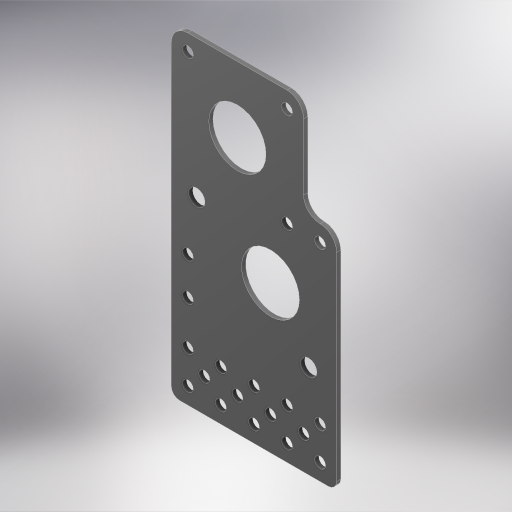
# Autodesk Inventor part: POM 1
Saved by Autodesk Inventor 2024 (Build 280153000, 153)
## iProperties
Created: 2023-09-01
Part Number: POM 1
Material: Acetal Resin, Black
Document SubType Name: Modeling
Designer: aaron
Density: 1.425 g/cm^3
Appearance: Smooth - Black
Author: aaron
Autodesk Inventor part; units mm, degrees
ref_plane "YZ Plane" through (0, 0, 0) normal (1, 0, 0) x (0, 1, 0)
ref_plane "XZ Plane" through (0, 0, 0) normal (0, 1, 0) x (-1, 0, 0)
ref_plane "XY Plane" through (0, 0, 0) normal (0, 0, 1) x (1, 0, 0)
sketch "Sketch1" plane through (0, 0, 0) normal (0, 0, 1) x (1, 0, 0)
  line L0 (57.15, -58.7375) -> (-57.15, -58.7375)
  line L1 (-57.15, -58.7375) -> (-57.15, 58.7375)
  line L2 (-57.15, 58.7375) -> (57.15, 58.7375)
  line L3 (57.15, 58.7375) -> (57.15, -58.7375)
  line L4 (57.15, -58.7375) -> (-57.15, 58.7375) construction
  line L5 (-57.15, -58.7375) -> (57.15, 58.7375) construction
  line L6 (-57.15, 58.7375) -> (-19.05, 58.7375)
  line L7 (-19.05, 58.7375) -> (-19.05, 20.6375)
  line L8 (-19.05, 20.6375) -> (-57.15, 20.6375)
  line L9 (-57.15, 20.6375) -> (-57.15, 58.7375)
  circle A0 centre (-38.1, 39.6875) radius 19.05
  circle A1 centre (-57.15, 58.7375) radius 6.35
  circle A2 centre (57.15, 58.7375) radius 6.35
  line L10 (-57.15, -58.7375) -> (-63.5, -58.7375)
  line L11 (-63.5, -58.7375) -> (-63.5, 58.7375)
  line L12 (57.15, -58.7375) -> (63.5, -58.7375)
  line L13 (63.5, -58.7375) -> (63.5, 58.7375)
  line L14 (57.15, 65.0875) -> (-57.15, 65.0875)
  circle A3 centre (-38.1, 39.6875) radius 10.9855
  circle A4 centre (-57.15, 58.7375) radius 2.1082
  circle A5 centre (57.15, 58.7375) radius 2.1082
  point P0 (0, 0)
  dimension "d0" = 114.3
  dimension "d1" = 117.475
  dimension "d2" = 38.1
  dimension "d3" = 38.1
  dimension "d4" = 12.7
  dimension "d5" = 12.7
  dimension "d8" = 21.971
  dimension "d9" = 4.2164
  dimension "d10" = 4.2164
  constraints: 30 end point, 6 centre point, 5 coincident, 4 horizontal, 4 parallel, 4 perpendicular, 4 point on circle, 3 tangent, 2 midpoint
  measures "d0" distance of L1.end L2.end
  measures "d1" distance of L0.end L1.end
  measures "d2" distance of L7.end L8.end
  measures "d3" distance of L6.end L7.end
  measures "d4" diameter of A1
  measures "d5" diameter of A2
  measures "d8" diameter of A3
  measures "d9" diameter of A4
  measures "d10" diameter of A5
extrude "Extrusion1" add sketch "Sketch1" along normal blind 1.5875 contours L0 L1 L8 L7 L2 A2 L3 | L3 A2 L13 L12 | L10 L11 A1 L1 | A2 L2 A5 L3 | L3 A5 L2 A2 | L1 A0 L8 | L2 A1 L14 A2 | L1 A1 L2 A0 | A0 | A0 L7 L8 | A1 L2 A4 L1 | L7 A0 L2 | L1 A4 L2 A1
sketch "Sketch2" plane through (0, 0, 1.5875) normal (0, 0, 1) x (1, 0, 0)
  circle A0 centre (-38.1, 39.6875) radius 10.9855 projected
  line L0 (-38.1, 39.6875) -> (63.5, 39.6875)
  line L1 (63.5, -58.7375) -> (63.5, 58.7375) projected
  circle A1 centre (-38.1, 39.6875) radius 6.35
  circle A2 centre (-12.7, 39.6875) radius 19.05
  circle A3 centre (38.1, 39.6875) radius 31.75
  circle A4 centre (-12.7, 39.6875) radius 10.9855
  circle A5 centre (38.1, 39.6875) radius 10.9855
  line L2 (-63.5, 58.7375) -> (-63.5, -58.7375) projected
  line L3 (-38.1, 39.6875) -> (-12.7, 39.6875)
  line L4 (57.15, 65.0875) -> (-57.15, 65.0875) projected
  line L5 (-63.5, -58.7375) -> (63.5, -58.7375) projected
  line L6 (0, -58.7375) -> (0, 65.0875)
  circle A6 centre (0, -46.0375) radius 19.05
  circle A7 centre (0, -46.0375) radius 2.1082
  point P0 (0, 0)
  dimension "d13" = 12.7
  dimension "d14" = 38.1
  dimension "d15" = 63.5
  dimension "d16" = 21.971
  dimension "d17" = 21.971
  dimension "d21" = 38.1
  dimension "d22" = 12.7
  dimension "d23" = 4.2164
  constraints: 7 centre point, 6 end point, 4 coincident, 4 point on line, 2 midpoint, 2 tangent, 1 collinear, 1 horizontal, 1 vertical
  measures "d13" diameter of A1
  measures "d14" diameter of A2
  measures "d15" diameter of A3
  measures "d16" diameter of A4
  measures "d17" diameter of A5
  measures "d21" diameter of A6
  measures "d22" distance from line of L5 A6.centre
  measures "d23" diameter of A7
extrude "Extrusion2" cut sketch "Sketch2" against normal blind 1.5875 contours A4 L0 | L0 A4 | A5 L0 | L0 A5 | A7 L6 | L6 A7
sketch "Sketch10" plane through (0, 0, 1.5875) normal (0, 0, 1) x (1, 0, 0)
  circle A0 centre (0, -46.0375) radius 2.1082 projected
  circle A1 centre (0, -46.0375) radius 19.05
  line L0 (0, -46.0375) -> (-10.7345, -23.0173)
  circle A2 centre (-10.7345, -23.0173) radius 6.35
  line L1 (57.15, 65.0875) -> (-57.15, 65.0875) projected
  line L2 (-63.5, -58.7375) -> (63.5, -58.7375) projected
  line L3 (0, -58.7375) -> (0, 65.0875)
  circle A3 centre (-25.4, -2.2788) radius 19.05
  line L4 (-25.4, 65.0875) -> (-25.4, -58.7375)
  circle A4 centre (-38.1, 39.6875) radius 10.9855 projected
  circle A5 centre (-38.1, 39.6875) radius 19.05
  circle A6 centre (-53.7317, 12.0522) radius 12.7
  point P0 (0, 0)
  dimension "d121" = 38.1
  dimension "d122" = 25.4
  dimension "d123" = 25
  dimension "d124" = 38.1
  dimension "d125" = 25.4
  dimension "d126" = 38.1
  dimension "d127" = 25.4
  constraints: 6 end point, 5 centre point, 4 tangent, 3 coincident, 3 point on line, 2 midpoint, 1 perpendicular
  measures "d121" diameter of A1
  measures "d122" distance of L0.start L0.end
  measures "d123" angle of L3 L0
  measures "d124" diameter of A3
  measures "d125" distance between parallel lines of L4 L3
  measures "d126" diameter of A5
  measures "d127" diameter of A6
sketch "Sketch11" plane through (0, 0, 1.5875) normal (0, 0, 1) x (1, 0, 0)
  circle A0 centre (-10.7345, -23.0173) radius 6.35 projected
  circle A1 centre (-25.4, -2.2788) radius 19.05 projected
  circle A2 centre (-53.7317, 12.0522) radius 12.7 projected
  circle A3 centre (-53.7317, 12.0522) radius 3.175
  circle A4 centre (-25.4, -2.2788) radius 3.9688
  circle A5 centre (-10.7345, -23.0173) radius 3.175
  point P0 (0, 0)
  dimension "d128" = 6.35
  dimension "d129" = 7.9375
  dimension "d130" = 6.35
  constraints: 3 centre point, 3 coincident
  measures "d128" diameter of A3
  measures "d129" diameter of A4
  measures "d130" diameter of A5
extrude "Extrusion9" cut sketch "Sketch11" against normal blind 25.4 contours A3 | A4 | A5
sketch "Sketch12" plane through (0, 0, 1.5875) normal (0, 0, 1) x (1, 0, 0)
  circle A0 centre (57.15, -52.3875) radius 2.1082
  circle A1 centre (0, -46.0375) radius 2.1082 projected
  line L0 (-63.5, -58.7375) -> (63.5, -58.7375) projected
  line L1 (-63.5, -58.7375) -> (63.5, -58.7375) projected
  line L2 (63.5, -58.7375) -> (63.5, 58.7375) projected
  circle A2 centre (44.45, -52.3875) radius 2.1082
  circle A3 centre (31.75, -52.3875) radius 2.1082
  circle A4 centre (19.05, -52.3875) radius 2.1082
  circle A5 centre (6.35, -52.3875) radius 2.1082
  circle A6 centre (-6.35, -52.3875) radius 2.1082
  circle A7 centre (-19.05, -52.3875) radius 2.1082
  circle A8 centre (-31.75, -52.3875) radius 2.1082
  circle A9 centre (-44.45, -52.3875) radius 2.1082
  circle A10 centre (-57.15, -52.3875) radius 2.1082
  circle A11 centre (57.15, -39.6875) radius 2.1082
  circle A12 centre (44.45, -39.6875) radius 2.1082
  circle A13 centre (31.75, -39.6875) radius 2.1082
  circle A14 centre (19.05, -39.6875) radius 2.1082
  circle A15 centre (6.35, -39.6875) radius 2.1082
  circle A16 centre (-6.35, -39.6875) radius 2.1082
  circle A17 centre (-19.05, -39.6875) radius 2.1082
  circle A18 centre (-31.75, -39.6875) radius 2.1082
  circle A19 centre (-44.45, -39.6875) radius 2.1082
  circle A20 centre (-57.15, -39.6875) radius 2.1082
  point P0 (0, 0)
  dimension "d133" = 4.2164
  dimension "d134" = 6.35
  dimension "d135" = 57.15
  dimension "d138" = 12.7
  dimension "d141" = 12.7
  constraints: 20 centre point, 1 horizontal, 1 vertical, 38 other
  measures "d133" diameter of A0
  measures "d134" vertical distance of A0.centre A1.centre
  measures "d135" horizontal distance of A1.centre A0.centre
  measures "d138" distance of A0.centre A2.centre
  measures "d141" distance of A0.centre A11.centre
extrude "Extrusion10" cut sketch "Sketch12" against normal blind 25.4
sketch "Sketch14" plane through (0, 0, 1.5875) normal (0, 0, 1) x (1, 0, 0)
  circle A0 centre (-25.4, -2.2788) radius 3.9687 projected
  circle A1 centre (-57.15, -8.6288) radius 2.1082
  line L0 (-63.5, 58.7375) -> (-63.5, -58.7375) projected
  line L1 (-63.5, -58.7375) -> (63.5, -58.7375) projected
  circle A2 centre (-57.15, 4.0712) radius 2.1082
  circle A3 centre (-44.45, -8.6288) radius 2.1082
  circle A4 centre (-44.45, 4.0712) radius 2.1082
  circle A5 centre (-31.75, -8.6288) radius 2.1082
  circle A6 centre (-31.75, 4.0712) radius 2.1082
  circle A7 centre (-19.05, -8.6288) radius 2.1082
  circle A8 centre (-19.05, 4.0712) radius 2.1082
  circle A9 centre (-6.35, -8.6288) radius 2.1082
  circle A10 centre (-6.35, 4.0712) radius 2.1082
  circle A11 centre (6.35, -8.6288) radius 2.1082
  circle A12 centre (6.35, 4.0712) radius 2.1082
  circle A13 centre (19.05, -8.6288) radius 2.1082
  circle A14 centre (19.05, 4.0712) radius 2.1082
  circle A15 centre (31.75, -8.6288) radius 2.1082
  circle A16 centre (31.75, 4.0712) radius 2.1082
  circle A17 centre (44.45, -8.6288) radius 2.1082
  circle A18 centre (44.45, 4.0712) radius 2.1082
  circle A19 centre (57.15, -8.6288) radius 2.1082
  circle A20 centre (57.15, 4.0712) radius 2.1082
  point P0 (0, 0)
  dimension "d159" = 4.2164
  dimension "d160" = 6.35
  dimension "d161" = 31.75
  dimension "d164" = 12.7
  dimension "d167" = 12.7
  constraints: 20 centre point, 1 horizontal, 1 vertical, 38 other
  measures "d159" diameter of A1
  measures "d160" vertical distance of A1.centre A0.centre
  measures "d161" horizontal distance of A0.centre A1.centre
  measures "d164" distance of A1.centre A2.centre
  measures "d167" distance of A1.centre A3.centre
extrude "Extrusion12" cut sketch "Sketch14" against normal blind 25.4 contours A0 | A1 | A2 | A3 | A4 | A5 | A6 | A7 | A8
sketch "Sketch16" plane through (0, 0, 1.5875) normal (0, 0, 1) x (1, 0, 0)
  circle A0 centre (-25.4, -2.2788) radius 2.1082
  circle A1 centre (0, -46.0375) radius 2.1082
  line L0 (-63.5, -58.7375) -> (63.5, -58.7375) projected
  circle A2 centre (12.7, -46.0375) radius 2.1082
  circle A3 centre (-12.7, -2.2788) radius 2.1082
  circle A4 centre (25.4, -46.0375) radius 2.1082
  circle A5 centre (0, -2.2788) radius 2.1082
  point P0 (0, 0)
  dimension "d185" = 4.2164
  dimension "d186" = 4.2164
  dimension "d189" = 12.7
  constraints: 6 centre point, 2 coincident, 1 horizontal, 8 other
  measures "d185" diameter of A0
  measures "d186" diameter of A1
  measures "d189" distance of A1.centre A2.centre
extrude "Extrusion14" cut sketch "Sketch16" against normal blind 25.4 contours A2 | A3 | A4 | A5
sketch "Sketch17" plane through (0, 0, 1.5875) normal (0, 0, 1) x (1, 0, 0)
  circle A0 centre (0, -46.0375) radius 2.1082
  circle A1 centre (-25.4, -2.2788) radius 2.1082
  line L0 (-63.5, 58.7375) -> (-63.5, -58.7375) projected
  circle A2 centre (0, -46.0375) radius 19.05 projected
  line L1 (-63.5, -58.7375) -> (63.5, -58.7375) projected
  circle A3 centre (-38.1, -2.2788) radius 2.1082
  circle A4 centre (-50.8, -2.2788) radius 2.1082
  circle A5 centre (-12.7, -2.2788) radius 2.1082
  circle A6 centre (-25.4, -2.2788) radius 2.1082
  circle A7 centre (-38.1, -2.2788) radius 2.1082
  circle A8 centre (0, -2.2788) radius 2.1082
  circle A9 centre (-12.7, -2.2788) radius 2.1082
  circle A10 centre (-25.4, -2.2788) radius 2.1082
  circle A11 centre (12.7, -2.2788) radius 2.1082
  circle A12 centre (0, -2.2788) radius 2.1082
  circle A13 centre (-12.7, -2.2788) radius 2.1082
  circle A14 centre (25.4, -2.2788) radius 2.1082
  circle A15 centre (12.7, -2.2788) radius 2.1082
  circle A16 centre (0, -2.2788) radius 2.1082
  circle A17 centre (38.1, -2.2788) radius 2.1082
  circle A18 centre (25.4, -2.2788) radius 2.1082
  circle A19 centre (12.7, -2.2788) radius 2.1082
  circle A20 centre (50.8, -2.2788) radius 2.1082
  circle A21 centre (38.1, -2.2788) radius 2.1082
  circle A22 centre (25.4, -2.2788) radius 2.1082
  circle A23 centre (12.7, -46.0375) radius 2.1082
  circle A24 centre (25.4, -46.0375) radius 2.1082
  circle A25 centre (38.1, -46.0375) radius 2.1082
  circle A26 centre (50.8, -46.0375) radius 2.1082
  circle A27 centre (-12.7, -46.0375) radius 2.1082
  circle A28 centre (0, -46.0375) radius 2.1082
  circle A29 centre (12.7, -46.0375) radius 2.1082
  circle A30 centre (25.4, -46.0375) radius 2.1082
  circle A31 centre (38.1, -46.0375) radius 2.1082
  circle A32 centre (-25.4, -46.0375) radius 2.1082
  circle A33 centre (-12.7, -46.0375) radius 2.1082
  circle A34 centre (0, -46.0375) radius 2.1082
  circle A35 centre (12.7, -46.0375) radius 2.1082
  circle A36 centre (25.4, -46.0375) radius 2.1082
  circle A37 centre (-38.1, -46.0375) radius 2.1082
  circle A38 centre (-25.4, -46.0375) radius 2.1082
  circle A39 centre (-12.7, -46.0375) radius 2.1082
  circle A40 centre (0, -46.0375) radius 2.1082
  circle A41 centre (12.7, -46.0375) radius 2.1082
  circle A42 centre (-50.8, -46.0375) radius 2.1082
  circle A43 centre (-38.1, -46.0375) radius 2.1082
  circle A44 centre (-25.4, -46.0375) radius 2.1082
  circle A45 centre (-12.7, -46.0375) radius 2.1082
  circle A46 centre (0, -46.0375) radius 2.1082
  point P0 (0, 0)
  dimension "d196" = 4.2164
  dimension "d197" = 4.2164
  dimension "d200" = 12.7
  dimension "d203" = 12.7
  dimension "d208" = 12.7
  dimension "d211" = 12.7
  constraints: 46 centre point, 4 horizontal, 2 coincident, 88 other
  measures "d196" diameter of A0
  measures "d197" diameter of A1
  measures "d200" distance of A1.centre A3.centre
  measures "d203" distance of A1.centre A5.centre
  measures "d208" distance of A0.centre A23.centre
  measures "d211" distance of A0.centre A27.centre
extrude "Extrusion15" cut sketch "Sketch17" against normal blind 25.4 contours A3 | A4 | A25 | A26 | A27 | A32 | A37 | A42
sketch "Sketch20" plane through (0, 0, 1.5875) normal (0, 0, 1) x (1, 0, 0)
  circle A0 centre (0, -2.2788) radius 2.1082 projected
  circle A1 centre (57.15, 33.3375) radius 2.1082 projected
  line L0 (57.15, 65.0875) -> (-57.15, 65.0875) projected
  line L1 (-63.5, -58.7375) -> (63.5, -58.7375) projected
  line L2 (6.35, -58.7375) -> (6.35, 65.0875)
  line L3 (63.5, -58.7375) -> (63.5, 58.7375) projected
  line L4 (0, -2.2788) -> (61.9125, -2.2788) construction
  circle A2 centre (31.75, -2.2788) radius 2.1082
  line L5 (31.75, -2.2788) -> (0, -2.2788)
  line L6 (31.75, -2.2788) -> (15.875, 25.2175)
  line L7 (0, -2.2788) -> (15.875, 25.2175)
  line L8 (15.875, 18.8675) -> (26.2507, 0.8962)
  line L9 (26.2507, 0.8962) -> (5.4993, 0.8962)
  line L10 (5.4993, 0.8962) -> (15.875, 18.8675)
  line L11 (5.4993, -5.4538) -> (26.2507, -5.4538)
  line L12 (26.2507, -5.4538) -> (15.875, -23.4251)
  line L13 (15.875, -23.4251) -> (5.4993, -5.4538)
  line L14 (21.3743, -26.6001) -> (31.75, -8.6288)
  line L15 (31.75, -8.6288) -> (42.1257, -26.6001)
  line L16 (42.1257, -26.6001) -> (21.3743, -26.6001)
  line L17 (47.625, -23.4251) -> (37.2493, -5.4538)
  line L18 (37.2493, -5.4538) -> (58.0007, -5.4538)
  line L19 (58.0007, -5.4538) -> (47.625, -23.4251)
  line L20 (58.0007, 0.8962) -> (37.2493, 0.8962)
  line L21 (37.2493, 0.8962) -> (47.625, 18.8675)
  line L22 (47.625, 18.8675) -> (58.0007, 0.8962)
  line L23 (42.1257, 22.0425) -> (31.75, 4.0712)
  line L24 (31.75, 4.0712) -> (21.3743, 22.0425)
  line L25 (21.3743, 22.0425) -> (42.1257, 22.0425)
  point P0 (0, 0)
  dimension "d240" = 6.35
  dimension "d242" = 4.2164
  dimension "d243" = 31.75
  dimension "d244" = 31.75
  dimension "d246" = 3.175
  dimension "d249" = 360
  dimension "d260" = 31.75
  constraints: 46 end point, 3 point on line, 1 centre point, 1 horizontal, 1 perpendicular, 39 other
  measures "d240" distance from line of L4.start L2
  measures "d242" diameter of A2
  measures "d243" distance of L5.start L5.end
  measures "d244" distance of L5.start L6.end
  measures "d246" distance between parallel lines of L6 L8
  measures "d260" distance of L4.start L5.start
extrude "Extrusion17" cut sketch "Sketch20" against normal blind 25.4 contours L11 L12 L13 L2 | L2 L13 L11 | L9 L10 L2 | L2 L10 L8 L9 | L5 L6 A2 | A2 L6 L5 | L14 L15 L16 | L17 L18 L19 | L20 L21 L22 | L23 L24 L25
fillet "Fillet2" radius 3.175 3 edges at (58.0007, -5.4538, 0.7937) (37.2493, -5.4538, 0.7937) (47.625, -23.4251, 0.7937)
pattern_circular "Circular Pattern2" count 6 over 360 about axis through (31.75, -2.2788, 1.5875) along (0, 0, -1) of "Fillet2"
sketch "Sketch21" plane through (0, 0, 1.5875) normal (0, 0, 1) x (1, 0, 0)
  circle A0 centre (31.75, -2.2788) radius 2.1082 projected
  circle A1 centre (57.15, 33.3375) radius 2.1082 projected
  circle A2 centre (6.35, -2.2788) radius 2.1082
  circle A3 centre (57.15, -2.2788) radius 2.1082
  circle A4 centre (0, -2.2788) radius 2.1082 projected
  point P0 (0, 0)
  dimension "d257" = 4.2164
  dimension "d258" = 4.2164
  dimension "d259" = 6.35
  constraints: 2 centre point
  measures "d257" diameter of A2
  measures "d258" diameter of A3
  measures "d259" distance of A4.centre A2.centre
extrude "Extrusion18" cut sketch "Sketch21" against normal blind 25.4 contours A2 | A3
sketch "Sketch22" plane through (0, 0, 1.5875) normal (0, 0, 1) x (1, 0, 0)
  circle A0 centre (-38.1, 39.6875) radius 10.9855 projected
  line L0 (-57.15, 20.6375) -> (-19.05, 20.6375)
  line L1 (-19.05, 20.6375) -> (-19.05, 58.7375)
  line L2 (-19.05, 58.7375) -> (-57.15, 58.7375)
  line L3 (-57.15, 58.7375) -> (-57.15, 20.6375)
  line L4 (-57.15, 20.6375) -> (-19.05, 58.7375) construction
  line L5 (-19.05, 20.6375) -> (-57.15, 58.7375) construction
  circle A1 centre (-19.05, 58.7375) radius 2.1082
  circle A2 centre (-19.05, 20.6375) radius 2.1082
  circle A3 centre (-53.7317, 12.0522) radius 3.175 projected
  circle A4 centre (-6.35, -39.6875) radius 2.1082 projected
  circle A5 centre (-57.15, 33.3375) radius 2.1082 projected
  circle A6 centre (-57.15, -23.0173) radius 2.1082
  circle A7 centre (-6.35, 20.6375) radius 2.1082
  circle A8 centre (-12.7, 39.6875) radius 10.9855 projected
  circle A9 centre (-12.7, 39.6875) radius 19.05
  circle A10 centre (-38.1, 39.6875) radius 19.05
  circle A11 centre (-10.7345, -23.0173) radius 3.175 projected
  circle A12 centre (-19.05, 4.0712) radius 2.1082 projected
  line L6 (-31.75, 20.6375) -> (6.35, 20.6375)
  line L7 (6.35, 20.6375) -> (6.35, 58.7375)
  line L8 (6.35, 58.7375) -> (-31.75, 58.7375)
  line L9 (-31.75, 58.7375) -> (-31.75, 20.6375)
  line L10 (-31.75, 20.6375) -> (6.35, 58.7375) construction
  line L11 (6.35, 20.6375) -> (-31.75, 58.7375) construction
  circle A13 centre (-12.7, 39.6875) radius 12.4333
  point P0 (0, 0)
  dimension "d264" = 38.1
  dimension "d265" = 4.2164
  dimension "d266" = 4.2164
  dimension "d267" = 4.2164
  dimension "d268" = 4.2164
  dimension "d269" = 38.1
  dimension "d270" = 38.1
  dimension "d271" = 0
  dimension "d274" = 38.1
  dimension "d275" = 38.1
  dimension "d276" = 24.8666
  dimension "d277" = 38.1
  constraints: 24 end point, 7 centre point, 5 coincident, 4 midpoint, 4 parallel, 2 horizontal, 2 perpendicular
  measures "d264" distance of L1.end L0.end
  measures "d265" diameter of A1
  measures "d266" diameter of A2
  measures "d267" diameter of A6
  measures "d268" diameter of A7
  measures "d269" diameter of A9
  measures "d270" diameter of A10
  measures "d271" vertical distance of A6.centre A11.centre
  measures "d274" distance of L8.end L7.end
  measures "d275" distance of L7.end L6.end
  measures "d276" diameter of A13
  measures "d277" distance between parallel lines of L3 L1
extrude "Extrusion19" cut sketch "Sketch22" against normal blind 25.4 contours A9 L1 A1 | A1 L2 L1 A9 | A9 L1 L0 A2 | A2 L1 A9 | A1 L8 L2 | L1 A9 A1 | L1 L8 A1 A9 | A2 A9 L1 | L0 L6 A2 | A9 A2 L6 L1 | A9 A7 L6 | A7 A9 | L6 A7 | A6 picked at (-6.6485, 20.9034)
fillet "Fillet3" radius 3.175 2 edges at (63.5, -58.7375, 0.7937) (-63.5, -58.7375, 0.7937)
sketch "Sketch23" plane through (0, 0, 1.5875) normal (0, 0, 1) x (1, 0, 0)
  circle A0 centre (-12.7, 39.6875) radius 10.9855 projected
  circle A1 centre (0, -46.0375) radius 2.1082 projected
  circle A2 centre (0, -2.2788) radius 2.1082 projected
  circle A3 centre (-12.7, -2.2788) radius 2.1082 projected
  circle A4 centre (-19.05, -8.6288) radius 2.1082 projected
  circle A5 centre (-31.75, -8.6288) radius 2.1082 projected
  circle A6 centre (-44.45, -8.6288) radius 2.1082 projected
  circle A7 centre (-57.15, -8.6288) radius 2.1082 projected
  circle A8 centre (-57.15, 4.0712) radius 2.1082 projected
  circle A9 centre (-50.8, -2.2788) radius 2.1082 projected
  circle A10 centre (-44.45, 4.0712) radius 2.1082 projected
  circle A11 centre (-38.1, -2.2788) radius 2.1082 projected
  circle A12 centre (-25.4, -2.2788) radius 3.9687 projected
  circle A13 centre (-31.75, 4.0712) radius 2.1082 projected
  circle A14 centre (-19.05, 4.0712) radius 2.1082 projected
  point P0 (0, 0)
extrude "Extrusion20" add sketch "Sketch23" against normal blind 1.5875 contours A0 | A1 | A2 | A3 | A4 | A5 | A6 | A8 | A9 | A10 | A11 | A12 | A13 | A14
sketch "Sketch24" plane through (0, 0, 1.5875) normal (0, 0, 1) x (1, 0, 0)
  circle A0 centre (-19.05, 58.7375) radius 2.1082 projected
  circle A1 centre (-19.05, 20.6375) radius 2.1082 projected
  circle A2 centre (-6.35, 20.6375) radius 2.1082 projected
  circle A3 centre (-19.05, 58.7375) radius 6.35
  line L0 (57.15, 65.0875) -> (-57.15, 65.0875) projected
  circle A4 centre (-6.35, 20.6375) radius 6.35
  circle A5 centre (-19.05, 20.6375) radius 6.35
  line L1 (-12.7, 58.7375) -> (-12.7, 20.6375)
  line L2 (-19.05, 26.9875) -> (-6.35, 26.9875)
  line L3 (0, 20.6375) -> (0, -60.8265)
  line L4 (-60.325, -58.7375) -> (60.325, -58.7375) projected
  arc A6 (60.325, -58.7375) -> (63.5, -55.5625) centre (60.325, -55.5625) ccw projected
  line L5 (63.5, -55.5625) -> (63.5, 58.7375) projected
  line L6 (57.15, 65.0875) -> (-57.15, 65.0875) projected
  arc A7 (63.5, 58.7375) -> (57.15, 65.0875) centre (57.15, 58.7375) ccw projected
  point P0 (0, 0)
  point P1 (-19.05, 65.0875)
  point P2 (-12.7, 26.9875)
  point P3 (0, -58.7375)
  dimension "d283" = 12.7
  dimension "d284" = 12.7
  constraints: 6 end point, 4 point on circle, 3 coincident, 2 centre point, 2 perpendicular, 1 horizontal, 1 tangent, 1 vertical, 3 other
  measures "d283" diameter of A4
  measures "d284" diameter of A5
extrude "Extrusion21" cut sketch "Sketch24" against normal blind 1.5875 contours A3 L0 A7 L5 A6 L4 L3 A4 L2 L1
fillet "Fillet4" radius 6.35 1 edges at (-12.7, 26.9875, 0.7937)
sketch "Sketch25" plane through (0, 0, 1.5875) normal (0, 0, 1) x (1, 0, 0)
  circle A0 centre (-53.7317, 12.0522) radius 3.175 projected
  circle A1 centre (-10.7345, -23.0173) radius 3.175 projected
  circle A2 centre (-25.4, -2.2788) radius 19.05 projected
  circle A3 centre (-25.4, -2.2788) radius 11.1125
  point P0 (0, 0)
  dimension "d288" = 22.225
  constraints: 1 centre point, 1 coincident
  measures "d288" diameter of A3
extrude "Extrusion22" cut sketch "Sketch25" against normal blind 1.5875 contours A3
fillet "Fillet5" radius 3.175 1 edges at (0, -58.7375, 0.7937)
body "Solid1"
